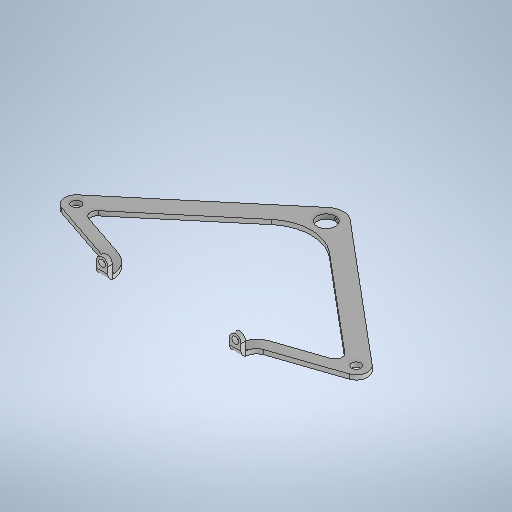
# Autodesk Inventor part: 01
Saved by Autodesk Inventor 2025.1 (Build 291241000, 241)
## iProperties
Created: 2024-09-13
Part Number: 01
Material: Generisch
Document SubType Name: Modeling
Designer: ffogue
Density: 1 g/cm^3
Appearance: Vorgabe
Author: ffogue
Autodesk Inventor part; units mm, degrees
note: some values were not read from the file. Chosen so that the rebuilt part matches the saved one: direction of "Hole2"; direction of "Hole3"; direction of "Hole4".
ref_plane "YZ Plane" through (0, 0, 0) normal (1, 0, 0) x (0, 1, 0)
sketch "Sketch1" plane through (0, 0, 0) normal (0, 0, 1) x (1, 0, 0)
  line L0 (-14.081, 0) -> (14.081, 0) construction
  line L1 (0, -22) -> (0, 22) construction
  arc A0 (12.8558, 37.3209) -> (-12.8558, 37.3209) centre (0, 22) ccw
  line L2 (-65.2139, 3.8302) -> (-4.8209, 54.5062)
  arc A1 (4.8209, 54.5062) -> (-4.8209, 54.5062) centre (0, 48.7609) ccw
  line L3 (4.8209, 54.5062) -> (65.2139, 3.8302)
  arc A2 (63.607, -4.7347) -> (65.2139, 3.8302) centre (62, 0) ccw
  line L4 (63.607, -4.7347) -> (35.393, -14.3106)
  arc A3 (35.393, -14.3106) -> (32, -19.0453) centre (37, -19.0453) ccw
  line L5 (32, -19.0453) -> (32, -21.0453) construction
  line L6 (27, -21.0453) -> (27, -19.0453) construction
  arc A4 (33.7861, -9.5759) -> (27, -19.0453) centre (37, -19.0453) ccw
  line L7 (33.7861, -9.5759) -> (53.6299, -2.8408)
  arc A5 (53.6299, -2.8408) -> (54.5941, 2.2981) centre (52.6657, 0) ccw
  line L8 (54.5941, 2.2981) -> (12.8558, 37.3209)
  line L9 (-12.8558, 37.3209) -> (-54.5941, 2.2981)
  arc A6 (-54.5941, 2.2981) -> (-53.6299, -2.8408) centre (-52.6657, 0) ccw
  line L10 (-53.6299, -2.8408) -> (-33.7861, -9.5759)
  arc A7 (-27, -19.0453) -> (-33.7861, -9.5759) centre (-37, -19.0453) ccw
  line L11 (-27, -19.0453) -> (-27, -21.0453) construction
  line L12 (-32, -21.0453) -> (-32, -19.0453) construction
  arc A8 (-32, -19.0453) -> (-35.393, -14.3106) centre (-37, -19.0453) ccw
  line L13 (-35.393, -14.3106) -> (-63.607, -4.7347)
  arc A9 (-65.2139, 3.8302) -> (-63.607, -4.7347) centre (-62, 0) ccw
  line L14 (-32, -19.0453) -> (-27, -19.0453)
  line L15 (32, -19.0453) -> (27, -19.0453)
  point P0 (0, 0)
  point P1 (0, 0)
  point P2 (-29.5, -21.0453)
  point P3 (29.5, -21.0453)
  dimension "d0" = 40
  dimension "d1" = 22
  dimension "d2" = 8
  dimension "d3" = 3
  dimension "d4" = 3
  dimension "d5" = 5
  dimension "d6" = 5
  dimension "d7" = 5
  dimension "d8" = 5
  dimension "d9" = 7.5
  dimension "d10" = 8
  dimension "d11" = 124
  dimension "d12" = 62
  dimension "d13" = 10
  dimension "d14" = 5
  dimension "d15" = 10
  dimension "d16" = 5
  dimension "d17" = 5
  dimension "d18" = 48.7609
  dimension "d20" = 29.5
  dimension "d21" = 59
  constraints: 32 end point, 20 point on circle, 18 tangent, 10 centre point, 7 horizontal alignment, 4 parallel, 3 vertical, 2 coincident, 2 midpoint, 1 horizontal, 1 vertical alignment
  measures "d0" diameter of A0
  measures "d1" distance of point (0, 0) L1.end
  measures "d2" distance between parallel lines of L3 L8
  measures "d3" radius of A5
  measures "d4" radius of A6
  measures "d5" radius of A9
  measures "d6" radius of A2
  measures "d7" distance of L11.end L12.start
  measures "d8" distance of L5.end L6.start
  measures "d9" radius of A1
  measures "d10" distance between parallel lines of L9 L2
  measures "d11" distance of A2.centre A9.centre
  measures "d12" distance of point (0, 0) A9.centre
  measures "d13" radius of A4
  measures "d14" radius of A3
  measures "d15" radius of A7
  measures "d16" radius of A8
  measures "d17" distance between parallel lines of L13 L10
  measures "d18" vertical distance of A1.centre A9.centre
  measures "d20" horizontal distance of point (0, 0) point (-29.5, -21.045)
  measures "d21" distance of point (29.5, -21.045) point (-29.5, -21.045)
extrude "Extrusion1" add sketch "Sketch1" along normal mid plane 2
ref_plane "Work Plane5" through (27, -19.0453, 1) normal (0, -1, 0) x (1, 0, 0)
sketch "Sketch5" plane through (27, -19.0453, 1) normal (0, -1, 0) x (1, 0, 0)
  line L0 (-54, -2) -> (-59, -2) projected
  line L1 (-54, -2) -> (-54, 0) projected
  line L2 (-59, 0) -> (-54, 0) projected
  line L3 (-59, -2) -> (-59, 0) projected
  line L4 (-54, -2) -> (-59, -2) projected
  line L5 (5, -2) -> (5, 0) projected
  line L6 (0, 0) -> (5, 0) projected
  line L7 (0, 0) -> (0, -2) projected
  line L8 (5, -2) -> (0, -2) projected
  line L9 (0, 0) -> (5, 0) projected
  line L10 (5, 0) -> (5, 4)
  arc A0 (5, 4) -> (0, 4) centre (2.5, 4) ccw
  line L11 (0, 4) -> (0, 0)
  line L12 (38.2139, 0) -> (-22.1791, 0) projected
  line L13 (-54, 0) -> (-54, 4)
  arc A1 (-54, 4) -> (-59, 4) centre (-56.5, 4) ccw
  line L14 (-59, 4) -> (-59, 0)
  point P0 (-27, -1)
  dimension "d29" = 2.5
  dimension "d30" = 2.5
  dimension "d31" = 4
  dimension "d32" = 4
  constraints: 8 end point, 4 point on circle, 4 tangent, 2 centre point, 2 vertical, 1 parallel, 1 perpendicular
  measures "d29" radius of A0
  measures "d30" radius of A1
  measures "d31" distance of L11.start L6.start
  measures "d32" distance of L1.end L13.end
extrude "Extrusion2" add sketch "Sketch5" along normal blind 2
fillet "Fillet3" radius 1 2 edges at (-29.5, -19.0453, 1) (29.5, -19.0453, 1)
fillet "Fillet4" radius 3 2 edges at (-29.5, -21.0453, -1) (29.5, -21.0453, -1)
sketch "Sketch7" plane through (27, -19.0453, 1) normal (0, 1, 0) x (1, 0, 0)
  arc A0 (-59, -4) -> (-54, -4) centre (-56.5, -4) ccw projected
  arc A1 (0, -4) -> (5, -4) centre (2.5, -4) ccw projected
  point P0 (-27, 1)
  constraints: 2 coincident
hole "Hole2" at (-29.5, -19.0453, 5) at (29.5, -19.0453, 5) direction (0, -1, 0) diameter 3 depth 2
sketch "Sketch8" plane through (0, 0, 1) normal (0, 0, 1) x (1, 0, 0)
  arc A0 (-65.2139, 3.8302) -> (-63.607, -4.7347) centre (-62, 0) ccw projected
  arc A1 (63.607, -4.7347) -> (65.2139, 3.8302) centre (62, 0) ccw projected
  point P0 (0, 0)
  constraints: 2 coincident
hole "Hole3" at (-62, 0, 1) at (62, 0, 1) direction (0, 0, -1) diameter 4 depth 2
sketch "Sketch9" plane through (0, 0, 1) normal (0, 0, 1) x (1, 0, 0)
  arc A0 (4.8209, 54.5062) -> (-4.8209, 54.5062) centre (0, 48.7609) ccw projected
  point P0 (0, 0)
  constraints: 1 coincident
hole "Hole4" at (0, 48.7609, 1) direction (0, 0, -1) diameter 8 depth 2
ref_plane "Work Plane6" through (0, 56.5, 0) normal (0, 1, 0) x (-1, 0, 0)
sketch "Sketch10" plane through (0, 56.5, 0) normal (0, 1, 0) x (-1, 0, 0)
  point P0 (0, 0)
  point P1 (0, 0)
  constraints: 1 coincident
hole "Hole5" at (0, 56.5, 0) direction (0, -1, 0) diameter 1 depth 4
equation "\"d4\" = d3"
equation "\"d6\" = d5"
equation "\"d10\" = d2"
equation "\"d12\" = 0.5 * d11"
equation "\"d15\" = d13"
equation "\"d16\" = d14"
equation "\"d21\" = 2 * d20"
equation "\"d32\" = d31"
body "Solid1"
